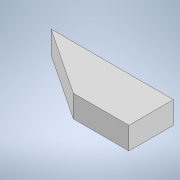
# Autodesk Inventor part: Slope
Saved by Autodesk Inventor 2021 (Build 250183000, 183)
## iProperties
Created: 2022-07-02
Part Number: Slope
Material: 一般
Document SubType Name: Modeling
Designer: tazak
Density: 1 g/cm^3
Appearance: 既定
Author: tazak
Autodesk Inventor part; units mm, degrees
ref_plane "YZ Plane" through (0, 0, 0) normal (1, 0, 0) x (0, 1, 0)
ref_plane "XZ Plane" through (0, 0, 0) normal (0, 1, 0) x (-1, 0, 0)
ref_plane "XY Plane" through (0, 0, 0) normal (0, 0, 1) x (1, 0, 0)
sketch "スケッチ1" plane through (0, 0, 0) normal (0, 0, 1) x (1, 0, 0)
  line L0 (5500, 1000) -> (11000, 1000)
  line L1 (11000, 1000) -> (11000, 0)
  line L2 (11000, 0) -> (5500, 0)
  line L3 (5500, 0) -> (5500, 1000)
  point P0 (0, 0)
  dimension "d13" = 5500
  dimension "d23" = 1000
  dimension "d24" = 5500
  constraints: 8 end point, 2 parallel, 1 horizontal, 1 horizontal alignment, 1 perpendicular
  measures "d13" distance of L0.start L0.end
  measures "d23" distance of L2.end L0.start
  measures "d24" distance from line of L3 point (0, 0)
extrude "押し出し1" add sketch "スケッチ1" along normal blind 2000
sketch "スケッチ5" plane through (5500, 0, 0) normal (0, -1, 0) x (1, 0, 0)
  line L0 (0, 0) -> (0, 2000) projected
  line L1 (0, 0) -> (3000, 2000)
  line L2 (0, 2000) -> (5500, 2000) projected
  point P0 (-5500, 0)
  dimension "d25" = 3000
  constraints: 2 end point, 1 point on line
  measures "d25" horizontal distance of L0.start L1.end
extrude "押し出し5" cut sketch "スケッチ5" against normal through all
